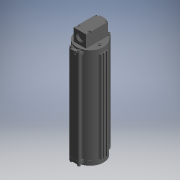
# Autodesk Inventor part: 1808236 DFPI-100-280-ND2P-E-P-G2(ZYL)
Saved by Autodesk Inventor 2017.3 (Build 213256000, 256)
## iProperties
Part Number: 1808236 DFPI-100-280-ND2P-E-P-G2(ZYL)
Material: Generic
Catalog Web Link: www.cadenas.de
Description: DFPI_ZYL-Linear drive - cylinder
Vendor: FESTO
Document SubType Name: Modeling
Designer: partserver
Manufacturer: FESTO
Mass: 1848.07 g
Surface Area: 3357.52 cm^2
Volume: 1848.07 cm^3
Density: 1 g/cm^3
Appearance: PSOLRGB-128-128-128
Category: PARTsolutions
Company: FESTO
Title: 1808236 DFPI-100-280-ND2P-E-P-G2(ZYL)
Author: Cadenas PARTsolutions
Comments: Linear drive - cylinder
PSOL_IDENT_0: {$CADENAS_DATA\23d-libs\festo\parts\d\dfpi\parts\dfpi_ep_zyl.prj},223 {VTYP=3D},{NB=1808236 DFPI-100
PSOL_IDENT_1: -280-ND2P-E-P-G2(ZYL)},{LINA=1808236 DFPI-100-280-ND2P-E-P-G2(ZYL)},{NN=DFPI_ZYL},{DATE=14.05.2021 0
PSOL_IDENT_2: 7:20:23},{GEOMDATE=12.05.2017 12:10:00},{VERSION=},{LINEID=260},{WBVAR=HUB},{WBNUMERIC=HUB}  {NB=180
PSOL_IDENT_3: 8236 DFPI-100-280-ND2P-E-P-G2(ZYL)},{LINA=1808236 DFPI-100-280-ND2P-E-P-G2(ZYL)},{KT=DUMMY},{TNR=180
PSOL_IDENT_4: 8236},{TYP=DFPI},{TYP2=DFPI-100-    -ND2P-E-P-G2},{HUB=280},{KDM=100},{DF=N},{WS=D2},{MF=P},{R=-},{R
PSOL_IDENT_5: 1=},{AR=E},{AR1=-E},{WV=-},{WV1=},{AF=P},{AF1=-P},{RM=-},{RM1=},{GEN=G2},{GEN1=-G2},{L0=118.500},{L0
PSOL_IDENT_6: 0=118.500},{L100=27.500},{X=0.000},{Y=0.000},{VERS=19}
NB: 1808236 DFPI-100-280-ND2P-E-P-G2(ZYL)
NN: DFPI_ZYL
NT: Linear drive - cylinder
NBSYN: $TNR. $TYP.-$KDM.-$HUB.-$DF.$WS.$MF.$R1.$AR1.$WV1.$AF1.$RM1.$GEN1.(ZYL)
LINA: 1808236 DFPI-100-280-ND2P-E-P-G2(ZYL)
CATALOG: Festo
TNR: 1808236
TYP: DFPI
TYP2: DFPI-100-    -ND2P-E-P-G2
HUB: 280
KDM: 100
DF: N
WS: D2
MF: P
R: -
AR: E
WV: -
AF: P
RM: -
GEN: G2
L0: 118.5
L00: 118.5
L100: 27.5
X: 0
Y: 0
VERS: 19
SUPPLIER: FESTO
ARTICLENO: 1808236 DFPI-100-280-ND2P-E-P-G2(ZYL)
BOMINFO: 1808236 DFPI-100-280-ND2P-E-P-G2(ZYL)
CREATOR: CADENAS GmbH
Autodesk Inventor part; units mm, degrees
sketch "Sketch_1" plane through (0, 0, 0) normal (0, 0, 1) x (1, 0, 0)
  arc A0 (-25.045, 47.8409) -> (-25.045, -47.8409) centre (0, 0) ccw
  arc A1 (-22.1168, -52.2342) -> (-25.045, -47.8409) centre (-27.5958, -52.7136) ccw
  line L0 (-22.1168, -52.2342) -> (-21.4753, -59.5665)
  arc A2 (-21.4753, -59.5665) -> (-15, -65.5) centre (-15, -59) ccw
  line L1 (-15, -65.5) -> (15, -65.5)
  arc A3 (15, -65.5) -> (21.4753, -59.5665) centre (15, -59) ccw
  line L2 (21.4753, -59.5665) -> (22.1168, -52.2342)
  arc A4 (25.045, -47.8409) -> (22.1168, -52.2342) centre (27.5958, -52.7136) ccw
  arc A5 (25.045, -47.8409) -> (25.045, 47.8409) centre (0, 0) ccw
  arc A6 (22.1168, 52.2342) -> (25.045, 47.8409) centre (27.5958, 52.7136) ccw
  line L3 (22.1168, 52.2342) -> (21.4753, 59.5665)
  arc A7 (21.4753, 59.5665) -> (15, 65.5) centre (15, 59) ccw
  line L4 (15, 65.5) -> (-15, 65.5)
  arc A8 (-15, 65.5) -> (-21.4753, 59.5665) centre (-15, 59) ccw
  line L5 (-21.4753, 59.5665) -> (-22.1168, 52.2342)
  arc A9 (-25.045, 47.8409) -> (-22.1168, 52.2342) centre (-27.5958, 52.7136) ccw
  constraints: 20 point on circle, 12 end point, 10 centre point
extrude "Extrusion1" add sketch "Sketch_1" against normal blind 19
sketch "Sketch_3" plane through (0, 0, -19) normal (0, 0, 1) x (1, 0, 0)
  arc A0 (-59.3893, 3.6277) -> (-59.3893, -3.6277) centre (0, 0) ccw
  line L0 (-59.3893, -3.6277) -> (-58.3519, -3.5187)
  arc A1 (-58.3519, -3.5187) -> (-58.1739, -3.2989) centre (-58.3728, -3.3198) ccw
  line L1 (-58.1739, -3.2989) -> (-58.2, -3.0503)
  arc A2 (-58.022, -2.8305) -> (-58.2, -3.0503) centre (-58.0011, -3.0294) ccw
  line L2 (-58.022, -2.8305) -> (-55.4362, -2.5587)
  arc A3 (-54.9966, -2.9147) -> (-55.4362, -2.5587) centre (-55.3944, -2.9565) ccw
  line L3 (-54.9966, -2.9147) -> (-54.4008, -8.5835)
  arc A4 (-54.7568, -9.0231) -> (-54.4008, -8.5835) centre (-54.7986, -8.6253) ccw
  line L4 (-54.7568, -9.0231) -> (-57.3426, -9.2948)
  arc A5 (-57.5624, -9.1168) -> (-57.3426, -9.2948) centre (-57.3635, -9.0959) ccw
  line L5 (-57.5624, -9.1168) -> (-57.5885, -8.8682)
  arc A6 (-57.5885, -8.8682) -> (-57.8083, -8.6902) centre (-57.7874, -8.8891) ccw
  line L6 (-57.8083, -8.6902) -> (-58.8458, -8.7993)
  arc A7 (-58.8458, -8.7993) -> (-58.2367, -12.1955) centre (0, 0) ccw
  arc A8 (-58.2367, -12.1955) -> (-58.0452, -12.46) centre (-57.8452, -12.1136) ccw
  line L7 (-58.0452, -12.46) -> (-52.7859, -15.4965)
  arc A9 (-50.1604, -18.606) -> (-52.7859, -15.4965) centre (-55.7859, -20.6926) ccw
  arc A10 (-50.1604, -18.606) -> (-20.8221, -49.2817) centre (0, 0) ccw
  arc A11 (-20.5042, -49.4958) -> (-20.8221, -49.2817) centre (-21.2113, -50.2029) ccw
  line L8 (-20.5042, -49.4958) -> (-17.7071, -52.2929)
  arc A12 (-17.7071, -53.7071) -> (-17.7071, -52.2929) centre (-18.4142, -53) ccw
  line L9 (-17.7071, -53.7071) -> (-21.0501, -57.0501)
  arc A13 (-21.0501, -57.0501) -> (-21.1657, -57.3678) centre (-20.7672, -57.3329) ccw
  line L10 (-21.1657, -57.3678) -> (-20.9772, -59.5229)
  arc A14 (-20.9772, -59.5229) -> (-15, -65) centre (-15, -59) ccw
  line L11 (-15, -65) -> (15, -65)
  arc A15 (15, -65) -> (20.9772, -59.5229) centre (15, -59) ccw
  line L12 (20.9772, -59.5229) -> (21.1657, -57.3678)
  arc A16 (21.1657, -57.3678) -> (21.0501, -57.0501) centre (20.7672, -57.3329) ccw
  line L13 (21.0501, -57.0501) -> (17.7071, -53.7071)
  arc A17 (17.7071, -52.2929) -> (17.7071, -53.7071) centre (18.4142, -53) ccw
  line L14 (17.7071, -52.2929) -> (20.5042, -49.4958)
  arc A18 (20.8221, -49.2817) -> (20.5042, -49.4958) centre (21.2113, -50.2029) ccw
  arc A19 (20.8221, -49.2817) -> (50.1604, -18.606) centre (0, 0) ccw
  arc A20 (52.7859, -15.4965) -> (50.1604, -18.606) centre (55.7859, -20.6926) ccw
  line L15 (52.7859, -15.4965) -> (58.0452, -12.46)
  arc A21 (58.0452, -12.46) -> (58.2367, -12.1955) centre (57.8452, -12.1136) ccw
  arc A22 (58.2367, -12.1955) -> (58.8458, -8.7993) centre (0, 0) ccw
  line L16 (58.8458, -8.7993) -> (57.8083, -8.6902)
  arc A23 (57.8083, -8.6902) -> (57.5885, -8.8682) centre (57.7874, -8.8891) ccw
  line L17 (57.5885, -8.8682) -> (57.5624, -9.1168)
  arc A24 (57.3426, -9.2948) -> (57.5624, -9.1168) centre (57.3635, -9.0959) ccw
  line L18 (57.3426, -9.2948) -> (54.7568, -9.0231)
  arc A25 (54.4008, -8.5835) -> (54.7568, -9.0231) centre (54.7986, -8.6253) ccw
  line L19 (54.4008, -8.5835) -> (54.9966, -2.9147)
  arc A26 (55.4362, -2.5587) -> (54.9966, -2.9147) centre (55.3944, -2.9565) ccw
  line L20 (55.4362, -2.5587) -> (58.022, -2.8305)
  arc A27 (58.2, -3.0503) -> (58.022, -2.8305) centre (58.0011, -3.0294) ccw
  line L21 (58.2, -3.0503) -> (58.1739, -3.2989)
  arc A28 (58.1739, -3.2989) -> (58.3519, -3.5187) centre (58.3728, -3.3198) ccw
  line L22 (58.3519, -3.5187) -> (59.3893, -3.6277)
  arc A29 (59.3893, -3.6277) -> (59.3893, 3.6277) centre (0, 0) ccw
  line L23 (59.3893, 3.6277) -> (58.3519, 3.5187)
  arc A30 (58.3519, 3.5187) -> (58.1739, 3.2989) centre (58.3728, 3.3198) ccw
  line L24 (58.1739, 3.2989) -> (58.2, 3.0503)
  arc A31 (58.022, 2.8305) -> (58.2, 3.0503) centre (58.0011, 3.0294) ccw
  line L25 (58.022, 2.8305) -> (55.4362, 2.5587)
  arc A32 (54.9966, 2.9147) -> (55.4362, 2.5587) centre (55.3944, 2.9565) ccw
  line L26 (54.9966, 2.9147) -> (54.4008, 8.5835)
  arc A33 (54.7568, 9.0231) -> (54.4008, 8.5835) centre (54.7986, 8.6253) ccw
  line L27 (54.7568, 9.0231) -> (57.3426, 9.2948)
  arc A34 (57.5624, 9.1168) -> (57.3426, 9.2948) centre (57.3635, 9.0959) ccw
  line L28 (57.5624, 9.1168) -> (57.5885, 8.8682)
  arc A35 (57.5885, 8.8682) -> (57.8083, 8.6902) centre (57.7874, 8.8891) ccw
  line L29 (57.8083, 8.6902) -> (58.8458, 8.7993)
  arc A36 (58.8458, 8.7993) -> (58.2367, 12.1955) centre (0, 0) ccw
  arc A37 (58.2367, 12.1955) -> (58.0452, 12.46) centre (57.8452, 12.1136) ccw
  line L30 (58.0452, 12.46) -> (52.7859, 15.4965)
  arc A38 (50.1604, 18.606) -> (52.7859, 15.4965) centre (55.7859, 20.6926) ccw
  arc A39 (50.1604, 18.606) -> (20.8221, 49.2817) centre (0, 0) ccw
  arc A40 (20.5042, 49.4958) -> (20.8221, 49.2817) centre (21.2113, 50.2029) ccw
  line L31 (20.5042, 49.4958) -> (17.7071, 52.2929)
  arc A41 (17.7071, 53.7071) -> (17.7071, 52.2929) centre (18.4142, 53) ccw
  line L32 (17.7071, 53.7071) -> (21.0501, 57.0501)
  arc A42 (21.0501, 57.0501) -> (21.1657, 57.3678) centre (20.7672, 57.3329) ccw
  line L33 (21.1657, 57.3678) -> (20.9772, 59.5229)
  arc A43 (20.9772, 59.5229) -> (15, 65) centre (15, 59) ccw
  line L34 (15, 65) -> (-15, 65)
  arc A44 (-15, 65) -> (-20.9772, 59.5229) centre (-15, 59) ccw
  line L35 (-20.9772, 59.5229) -> (-21.1657, 57.3678)
  arc A45 (-21.1657, 57.3678) -> (-21.0501, 57.0501) centre (-20.7672, 57.3329) ccw
  line L36 (-21.0501, 57.0501) -> (-17.7071, 53.7071)
  arc A46 (-17.7071, 52.2929) -> (-17.7071, 53.7071) centre (-18.4142, 53) ccw
  line L37 (-17.7071, 52.2929) -> (-20.5042, 49.4958)
  arc A47 (-20.8221, 49.2817) -> (-20.5042, 49.4958) centre (-21.2113, 50.2029) ccw
  arc A48 (-20.8221, 49.2817) -> (-50.1604, 18.606) centre (0, 0) ccw
  arc A49 (-52.7859, 15.4965) -> (-50.1604, 18.606) centre (-55.7859, 20.6926) ccw
  line L38 (-52.7859, 15.4965) -> (-58.0452, 12.46)
  arc A50 (-58.0452, 12.46) -> (-58.2367, 12.1955) centre (-57.8452, 12.1136) ccw
  arc A51 (-58.2367, 12.1955) -> (-58.8458, 8.7993) centre (0, 0) ccw
  line L39 (-58.8458, 8.7993) -> (-57.8083, 8.6902)
  arc A52 (-57.8083, 8.6902) -> (-57.5885, 8.8682) centre (-57.7874, 8.8891) ccw
  line L40 (-57.5885, 8.8682) -> (-57.5624, 9.1168)
  arc A53 (-57.3426, 9.2948) -> (-57.5624, 9.1168) centre (-57.3635, 9.0959) ccw
  line L41 (-57.3426, 9.2948) -> (-54.7568, 9.0231)
  arc A54 (-54.4008, 8.5835) -> (-54.7568, 9.0231) centre (-54.7986, 8.6253) ccw
  line L42 (-54.4008, 8.5835) -> (-54.9966, 2.9147)
  arc A55 (-55.4362, 2.5587) -> (-54.9966, 2.9147) centre (-55.3944, 2.9565) ccw
  line L43 (-55.4362, 2.5587) -> (-58.022, 2.8305)
  arc A56 (-58.2, 3.0503) -> (-58.022, 2.8305) centre (-58.0011, 3.0294) ccw
  line L44 (-58.2, 3.0503) -> (-58.1739, 3.2989)
  arc A57 (-58.1739, 3.2989) -> (-58.3519, 3.5187) centre (-58.3728, 3.3198) ccw
  line L45 (-58.3519, 3.5187) -> (-59.3893, 3.6277)
  constraints: 116 point on circle, 92 end point, 58 centre point
extrude "Extrusion2" add sketch "Sketch_3" against normal blind 362
sketch "Sketch_4" plane through (0, 0, -381) normal (0, 0, 1) x (1, 0, 0)
  arc A0 (-25.045, 47.8409) -> (-25.045, -47.8409) centre (0, 0) ccw
  arc A1 (-22.1168, -52.2342) -> (-25.045, -47.8409) centre (-27.5958, -52.7136) ccw
  line L0 (-22.1168, -52.2342) -> (-21.4753, -59.5665)
  arc A2 (-21.4753, -59.5665) -> (-15, -65.5) centre (-15, -59) ccw
  line L1 (-15, -65.5) -> (15, -65.5)
  arc A3 (15, -65.5) -> (21.4753, -59.5665) centre (15, -59) ccw
  line L2 (21.4753, -59.5665) -> (22.1168, -52.2342)
  arc A4 (25.045, -47.8409) -> (22.1168, -52.2342) centre (27.5958, -52.7136) ccw
  arc A5 (25.045, -47.8409) -> (25.045, 47.8409) centre (0, 0) ccw
  arc A6 (22.1168, 52.2342) -> (25.045, 47.8409) centre (27.5958, 52.7136) ccw
  line L3 (22.1168, 52.2342) -> (21.4753, 59.5665)
  arc A7 (21.4753, 59.5665) -> (15, 65.5) centre (15, 59) ccw
  line L4 (15, 65.5) -> (-15, 65.5)
  arc A8 (-15, 65.5) -> (-21.4753, 59.5665) centre (-15, 59) ccw
  line L5 (-21.4753, 59.5665) -> (-22.1168, 52.2342)
  arc A9 (-25.045, 47.8409) -> (-22.1168, 52.2342) centre (-27.5958, 52.7136) ccw
  constraints: 20 point on circle, 12 end point, 10 centre point
extrude "Extrusion3" add sketch "Sketch_4" against normal blind 17.5
sketch "Sketch_5" plane through (0, 0, 0) normal (1, 0, 0) x (0, 1, 0)
  line L0 (0, -398.5) -> (0, 0)
  line L1 (54, 0) -> (54, -6.5)
  line L2 (54, -6.5) -> (69, -6.5)
  line L3 (69, -6.5) -> (69, -392)
  line L4 (69, -392) -> (54, -392)
  line L5 (54, -392) -> (54, -398.5)
  line L6 (54, -398.5) -> (70, -398.5)
  line L7 (70, -398.5) -> (70, 0)
  line L8 (70, 0) -> (54, 0)
  constraints: 18 end point
revolve "Revolution1" cut sketch "Sketch_5" angle 360 about axis through (0, 0, -398.5) along (0, 0, -1)
sketch "Sketch_2" plane through (15, 0, 0) normal (1, 0, 0) x (0, 0, -1)
  line L0 (6.5, 59) -> (-0.7, 59)
  line L1 (3.7434, 59) -> (2.3, 61.5)
  line L2 (2.3, 61.5) -> (-0.2, 61.5)
  line L3 (-0.2, 61.5) -> (-0.7, 62)
  line L4 (-0.7, 62) -> (-0.7, 63.4)
  line L5 (-0.7, 63.4) -> (-0.1, 64)
  line L6 (-0.1, 64) -> (5, 64)
  line L7 (5, 64) -> (5.3, 63.7)
  line L8 (5.3, 63.7) -> (5.3, 65.1)
  line L9 (5.3, 65.1) -> (6.5, 65.1)
  line L10 (6.5, 65.1) -> (6.5, 59)
  line L11 (6.5, 59) -> (3.7434, 59)
  constraints: 24 end point
revolve "Revolution2" add sketch "Sketch_2" angle 360 about axis through (15, 59, -6.5) along (0, 0, -1)
sketch "Sketch_6" plane through (0, 0, 0.7) normal (0, 0, 1) x (1, 0, 0)
  line L0 (12.5, 57.5566) -> (15, 56.1132)
  line L1 (15, 56.1132) -> (17.5, 57.5566)
  line L2 (17.5, 57.5566) -> (17.5, 60.4434)
  line L3 (17.5, 60.4434) -> (15, 61.8868)
  line L4 (15, 61.8868) -> (12.5, 60.4434)
  line L5 (12.5, 60.4434) -> (12.5, 57.5566)
  constraints: 12 end point
extrude "Extrusion4" cut sketch "Sketch_6" against normal blind 3
pattern_linear "Rectangular Pattern1" count 2 spacing 30 along (-1, 0, 0) count 2 spacing 118 along (0, -1, 0) of "Revolution2"
pattern_linear "Rectangular Pattern2" count 2 spacing 30 along (-1, 0, 0) count 2 spacing 118 along (0, -1, 0) of "Extrusion4"
sketch "Sketch_10" plane through (0, 0, -398.3) normal (0, 0, 1) x (1, 0, 0)
  arc A0 (-26, -35.7946) -> (-23.5301, -40.1071) centre (-21, -35.7946) ccw
  arc A1 (-23.5301, -40.1071) -> (23.5301, -40.1071) centre (0, 0) ccw
  arc A2 (23.5301, -40.1071) -> (26, -35.7946) centre (21, -35.7946) ccw
  line L0 (26, -35.7946) -> (26, 55)
  line L1 (26, 55) -> (-26, 55)
  line L2 (-26, 55) -> (-26, -35.7946)
  constraints: 6 end point, 6 point on circle, 3 centre point
extrude "Extrusion5" cut sketch "Sketch_10" against normal blind 0.2
sketch "Sketch_16" plane through (0, 0, -386.5) normal (0, 0, 1) x (1, 0, 0)
  line L0 (-11.8262, -71.0631) -> (-2.7631, -75.2893)
  line L1 (-2.7631, -75.2893) -> (1.4631, -66.2262)
  line L2 (1.4631, -66.2262) -> (-7.6, -62)
  line L3 (-7.6, -62) -> (-11.8262, -71.0631)
  constraints: 8 end point
extrude "Extrusion6" cut sketch "Sketch_16" along normal mid plane 11
sketch "Sketch_11" plane through (15, 0, 0) normal (1, 0, 0) x (0, 0, -1)
  line L0 (399.2, 59) -> (392, 59)
  line L1 (392, 59) -> (392, 65.1)
  line L2 (392, 65.1) -> (393.2, 65.1)
  line L3 (393.2, 65.1) -> (393.2, 63.7)
  line L4 (393.2, 63.7) -> (393.5, 64)
  line L5 (393.5, 64) -> (398.6, 64)
  line L6 (398.6, 64) -> (399.2, 63.4)
  line L7 (399.2, 63.4) -> (399.2, 62)
  line L8 (399.2, 62) -> (398.7, 61.5)
  line L9 (398.7, 61.5) -> (396.2, 61.5)
  line L10 (396.2, 61.5) -> (394.7566, 59)
  line L11 (394.7566, 59) -> (392, 59)
  constraints: 24 end point
revolve "Revolution3" add sketch "Sketch_11" angle 360 about axis through (15, 59, -399.2) along (0, 0, -1)
pattern_linear "Rectangular Pattern3" count 2 spacing 30 along (-1, 0, 0) count 2 spacing 118 along (0, -1, 0) of "Revolution3"
sketch "Sketch_13" plane through (0, 0, -399.2) normal (0, 0, 1) x (1, 0, 0)
  line L0 (12.5, 57.5566) -> (15, 56.1132)
  line L1 (15, 56.1132) -> (17.5, 57.5566)
  line L2 (17.5, 57.5566) -> (17.5, 60.4434)
  line L3 (17.5, 60.4434) -> (15, 61.8868)
  line L4 (15, 61.8868) -> (12.5, 60.4434)
  line L5 (12.5, 60.4434) -> (12.5, 57.5566)
  constraints: 12 end point
extrude "Extrusion7" cut sketch "Sketch_13" along normal blind 3
pattern_linear "Rectangular Pattern4" count 2 spacing 30 along (-1, 0, 0) count 2 spacing 118 along (0, -1, 0) of "Extrusion7"
sketch "Sketch11" plane through (0, 0, 0) normal (0, 0, 1) x (1, 0, 0)
  point P0 (24.7487, 24.7487)
hole "Hole1" at (24.7487, 24.7487, 0) direction (0, 0, -1) diameter 6.647 depth 19 tip angle 120 countersink diameter 8 countersink angle 90 thread size "M8x1.25" class "6H" standard "ISO Metric profile"
pattern_linear "Rectangular Pattern5" count 2 spacing 49.4975 along (-1, 0, 0) count 2 spacing 49.4975 along (0, -1, 0) of "Hole1"
sketch "Sketch_19" plane through (0, 0, 0) normal (0, 1, 0) x (-1, 0, 0)
  line L0 (40, -403.2) -> (40, -398.5)
  line L1 (40, -398.5) -> (45.1, -398.5)
  line L2 (45.1, -398.5) -> (45.1, -399.5)
  line L3 (45.1, -399.5) -> (44.75, -399.5)
  line L4 (44.75, -399.5) -> (44.75, -402.0616)
  arc A0 (44.6291, -402.2453) -> (44.75, -402.0616) centre (44.55, -402.0616) ccw
  arc A1 (40, -403.2) -> (44.6291, -402.2453) centre (40, -391.5) ccw
  line L5 (40, -403.2) -> (40, -398.5)
  constraints: 12 end point, 4 point on circle, 2 centre point
revolve "Revolution4" add sketch "Sketch_19" angle 360 about axis through (-40, 0, -403.2) along (0, 0, -1)
sketch "Sketch_20" plane through (0, 0, -403.2) normal (0, 0, 1) x (1, 0, 0)
  line L0 (-42.45, -0.6125) -> (-40.98, -0.4839)
  line L1 (-40.98, -0.4839) -> (-40.6125, -0.6125)
  line L2 (-40.6125, -0.6125) -> (-40.4839, -0.98)
  line L3 (-40.4839, -0.98) -> (-40.6125, -2.45)
  line L4 (-40.6125, -2.45) -> (-39.3875, -2.45)
  line L5 (-39.3875, -2.45) -> (-39.5161, -0.98)
  line L6 (-39.5161, -0.98) -> (-39.3875, -0.6125)
  line L7 (-39.3875, -0.6125) -> (-39.02, -0.4839)
  line L8 (-39.02, -0.4839) -> (-37.55, -0.6125)
  line L9 (-37.55, -0.6125) -> (-37.55, 0.6125)
  line L10 (-37.55, 0.6125) -> (-39.02, 0.4839)
  line L11 (-39.02, 0.4839) -> (-39.3875, 0.6125)
  line L12 (-39.3875, 0.6125) -> (-39.5161, 0.98)
  line L13 (-39.5161, 0.98) -> (-39.3875, 2.45)
  line L14 (-39.3875, 2.45) -> (-40.6125, 2.45)
  line L15 (-40.6125, 2.45) -> (-40.4839, 0.98)
  line L16 (-40.4839, 0.98) -> (-40.6125, 0.6125)
  line L17 (-40.6125, 0.6125) -> (-40.98, 0.4839)
  line L18 (-40.98, 0.4839) -> (-42.45, 0.6125)
  line L19 (-42.45, 0.6125) -> (-42.45, -0.6125)
  constraints: 40 end point
extrude "Extrusion8" cut sketch "Sketch_20" along normal blind 3
sketch "Sketch_22" plane through (0, 0, -398.5) normal (0, 0, 1) x (1, 0, 0)
  line L0 (-43, -17.8) -> (-37, -17.8)
  line L1 (-37, -17.8) -> (-37, -9)
  line L2 (-37, -9) -> (-43, -9)
  line L3 (-43, -9) -> (-43, -17.8)
  constraints: 8 end point
extrude "Extrusion9" cut sketch "Sketch_22" along normal blind 0.1
sketch "Sketch_21" plane through (0, 0, -398.5) normal (0, 0, 1) x (1, 0, 0)
  line L0 (-43, -17.8) -> (-37, -17.8)
  line L1 (-37, -17.8) -> (-37, -9)
  line L2 (-37, -9) -> (-43, -9)
  line L3 (-43, -9) -> (-43, -17.8)
  line L4 (-41, -16.8) -> (-39, -16.8)
  line L5 (-39, -16.8) -> (-39, -16.7)
  line L6 (-39, -16.7) -> (-41, -16.7)
  line L7 (-41, -16.7) -> (-41, -16.8)
  line L8 (-41.75, -15.4) -> (-38.25, -15.4)
  line L9 (-38.25, -15.4) -> (-38.25, -15.3)
  line L10 (-38.25, -15.3) -> (-41.75, -15.3)
  line L11 (-41.75, -15.3) -> (-41.75, -15.4)
  line L12 (-42.5, -13.9) -> (-42.5, -14)
  line L13 (-42.5, -14) -> (-37.5, -14)
  line L14 (-37.5, -14) -> (-37.5, -13.9)
  line L15 (-37.5, -13.9) -> (-39.95, -13.9)
  line L16 (-39.95, -13.9) -> (-39.95, -10)
  line L17 (-39.95, -10) -> (-40.05, -10)
  line L18 (-40.05, -10) -> (-40.05, -13.9)
  line L19 (-40.05, -13.9) -> (-42.5, -13.9)
  constraints: 40 end point
extrude "Extrusion10" add sketch "Sketch_21" along normal blind 1
sketch "Sketch_7" plane through (0, 0, -398.3) normal (0, 0, 1) x (1, 0, 0)
  line L0 (-24.5, 46.8802) -> (-24.5, -40.25)
  line L1 (-24.5, -40.25) -> (24.5, -40.25)
  line L2 (24.5, -40.25) -> (24.5, 46.8802)
  arc A0 (24.5, 46.8802) -> (23.3654, 48.6832) centre (22.5, 46.8802) ccw
  arc A1 (23.3654, 48.6832) -> (-23.3654, 48.6832) centre (0, 0) ccw
  arc A2 (-23.3654, 48.6832) -> (-24.5, 46.8802) centre (-22.5, 46.8802) ccw
  constraints: 6 end point, 6 point on circle, 3 centre point
extrude "Extrusion11" add sketch "Sketch_7" against normal blind 49
sketch "Sketch_24" plane through (0, 0, -447.3) normal (0, 0, 1) x (1, 0, 0)
  line L0 (-35, -30.5) -> (-20.25, -30.5)
  arc A0 (-20.25, -30.5) -> (-20.25, -20.5) centre (-20.25, -25.5) ccw
  line L1 (-20.25, -20.5) -> (-33, -20.5)
  line L2 (-33, -20.5) -> (-33, 40)
  line L3 (-33, 40) -> (-20.25, 40)
  arc A1 (-20.25, 40) -> (-15.25, 45) centre (-20.25, 45) ccw
  line L4 (-15.25, 45) -> (-15.25, 56.5)
  line L5 (-15.25, 56.5) -> (15.25, 56.5)
  line L6 (15.25, 56.5) -> (15.25, 45)
  arc A2 (15.25, 45) -> (20.25, 40) centre (20.25, 45) ccw
  line L7 (20.25, 40) -> (33, 40)
  line L8 (33, 40) -> (33, -20.5)
  line L9 (33, -20.5) -> (20.25, -20.5)
  arc A3 (20.25, -20.5) -> (20.25, -30.5) centre (20.25, -25.5) ccw
  line L10 (20.25, -30.5) -> (35, -30.5)
  line L11 (35, -30.5) -> (35, 59.5)
  line L12 (35, 59.5) -> (-35, 59.5)
  line L13 (-35, 59.5) -> (-35, -30.5)
  constraints: 28 end point, 8 point on circle, 4 centre point
extrude "Extrusion12" cut sketch "Sketch_24" along normal blind 5.4
sketch "Sketch_25" plane through (-20.25, 0, 0) normal (1, 0, 0) x (0, 0, -1)
  line L0 (446.9, 45) -> (441.9, 45)
  line L1 (441.9, 45) -> (441.9, 49.25)
  line L2 (441.9, 49.25) -> (446.4, 49.25)
  line L3 (446.4, 49.25) -> (446.9, 48.75)
  line L4 (446.9, 48.75) -> (446.9, 47.4)
  line L5 (446.9, 47.4) -> (446.5, 47)
  line L6 (446.5, 47) -> (444.4, 47)
  line L7 (444.4, 47) -> (443.2453, 45)
  line L8 (443.2453, 45) -> (441.9, 45)
  constraints: 18 end point
revolve "Revolution5" add sketch "Sketch_25" angle 360 about axis through (-20.25, 45, -446.9) along (0, 0, -1)
pattern_linear "Rectangular Pattern6" count 2 spacing 40.5 along (1, 0, 0) count 2 spacing 70.5 along (0, -1, 0) of "Revolution5"
sketch "Sketch_27" plane through (0, 0, -446.9) normal (0, 0, 1) x (1, 0, 0)
  line L0 (-22.25, 43.8453) -> (-20.25, 42.6906)
  line L1 (-20.25, 42.6906) -> (-18.25, 43.8453)
  line L2 (-18.25, 43.8453) -> (-18.25, 46.1547)
  line L3 (-18.25, 46.1547) -> (-20.25, 47.3094)
  line L4 (-20.25, 47.3094) -> (-22.25, 46.1547)
  line L5 (-22.25, 46.1547) -> (-22.25, 43.8453)
  constraints: 12 end point
extrude "Extrusion13" cut sketch "Sketch_27" along normal blind 2.5
pattern_linear "Rectangular Pattern7" count 2 spacing 40.5 along (1, 0, 0) count 2 spacing 70.5 along (0, -1, 0) of "Extrusion13"
sketch "Sketch_33" plane through (0, 0, 0) normal (1, 0, 0) x (0, 1, 0)
  line L0 (-29.25, -424.5) -> (-40.25, -424.5)
  line L1 (-40.25, -424.5) -> (-40.25, -408.5)
  line L2 (-40.25, -408.5) -> (-39.1675, -409.5825)
  line L3 (-39.1675, -409.5825) -> (-30.3325, -409.5825)
  line L4 (-30.3325, -409.5825) -> (-29.25, -408.5)
  line L5 (-29.25, -408.5) -> (-29.25, -424.5)
  line L6 (-29.25, -424.5) -> (-40.25, -424.5)
  constraints: 14 end point
revolve "Revolution6" cut sketch "Sketch_33" angle 360 about axis through (0, -29.25, -424.5) along (0, 1, 0)
thread "Thread1" size "M32x2" class "6H" standard "ISO Metric profile" full length
sketch "Sketch_32" plane through (0, 0, 0) normal (1, 0, 0) x (0, 1, 0)
  line L0 (0, -371) -> (0, 0)
  line L1 (0, 0) -> (12.5, 0)
  line L2 (12.5, 0) -> (12.5, -66)
  line L3 (12.5, -66) -> (50, -66)
  line L4 (50, -66) -> (50, -371)
  line L5 (50, -371) -> (0, -371)
  line L6 (0, -371) -> (0, 0)
  constraints: 14 end point
revolve "Revolution7" cut sketch "Sketch_32" angle 360 about axis through (0, 0, -371) along (0, 0, -1)
ref_plane "TO_DUMMY_XY" through (0, 0, 0) normal (0, 0, 1) x (1, 0, 0)
ref_plane "TO_DUMMY_YZ" through (0, 0, 0) normal (1, 0, 0) x (0, 1, 0)
ref_plane "TO_DUMMY_ZX" through (0, 0, 0) normal (0, 1, 0) x (0, 0, 1)
ref_plane "TO_KOLBEN_XY" through (0, 0, -371) normal (0, 0, 1) x (1, 0, 0)
ref_plane "TO_KOLBEN_YZ" through (0, 0, -371) normal (1, 0, 0) x (0, 1, 0)
ref_plane "TO_KOLBEN_ZX" through (0, 0, -371) normal (0, 1, 0) x (0, 0, 1)
body "Solid1"
